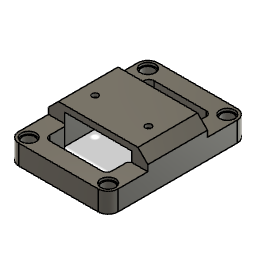
крепление двигателя (Autodesk Fusion 360 design; units mm, degrees)
Autodesk Fusion 360 part; units mm, degrees
sketch "Sketch1" plane through (0, 0, 0) normal (0, 1, 0) x (1, 0, 0)
  line L0 (-16, 24) -> (16, 24)
  line L1 (16, 24) -> (16, -24)
  line L2 (16, -24) -> (-16, -24)
  line L3 (-16, -24) -> (-16, 24)
  line L4 (-16, 24) -> (16, -24) construction
  line L5 (16, 24) -> (-16, -24) construction
  line L6 (-20, 28) -> (20, 28)
  line L7 (20, 28) -> (20, -28)
  line L8 (20, -28) -> (-20, -28)
  line L9 (-20, -28) -> (-20, 28)
  line L10 (-20, 28) -> (20, -28) construction
  line L11 (20, 28) -> (-20, -28) construction
  circle A0 centre (-16, 24) radius 2.5
  circle A1 centre (16, 24) radius 2.5
  circle A2 centre (-16, -24) radius 2.5
  circle A3 centre (16, -24) radius 2.5
  circle A4 centre (16, 24) radius 4
  circle A5 centre (-16, 24) radius 4
  circle A6 centre (-16, -24) radius 4
  circle A7 centre (16, -24) radius 4
  dimension "d1" = 32
  dimension "d2" = 48
  dimension "d3" = 40
  dimension "d4" = 56
  dimension "d5" = 5
  dimension "d6" = 5
  dimension "d7" = 5
  dimension "d8" = 5
  constraint horizontal L0
  constraint perpendicular L0 L1
  constraint parallel L0 L2
  constraint parallel L1 L3
  constraint coincident L4 origin
  constraint coincident L5 origin
  constraint horizontal L6
  constraint perpendicular L6 L7
  constraint parallel L6 L8
  constraint parallel L7 L9
  constraint coincident L10 origin
  constraint coincident L11 origin
  constraint coincident L0.start L3.end
  constraint coincident L0.end L1.start
  constraint coincident L2.end L3.start
  constraint coincident L1.end L2.start
  constraint concentric A1 A4
  constraint tangent L6 A4
  constraint concentric A0 A5
  constraint tangent L6 A5
  constraint concentric A2 A6
  constraint tangent L9 A6
  constraint concentric A3 A7
  constraint tangent L7 A7
  measures "d1" distance of L1.end L2.end
  measures "d2" distance of L0.end L1.end
  measures "d3" distance of L7.end L8.end
  measures "d4" distance of L6.end L7.end
  measures "d5" diameter of A0
  measures "d6" diameter of A1
  measures "d7" diameter of A2
  measures "d8" diameter of A3
extrude "Extrude1" add sketch "Sketch1" along normal blind 2.5 contours L0 L3 A0 A5 | L0 L3 A0 A5 | L0 L6 A4 A5 | L0 L1 L2 L3 A4 A5 A6 A7 | L3 L9 A5 A6 | L0 L1 A1 A4 | L0 L1 A1 A4 | L2 L3 A2 A6 | L2 L3 A2 A6 | L1 L7 A4 A7 | L2 L8 A6 A7 | L1 L2 A3 A7 | L1 L2 A3 A7 makes body 1
sketch "Sketch2" plane through (0, 2.5, 0) normal (0, 1, 0) x (-1, 0, 0)
  circle A0 centre (16, 24) radius 2.5
  circle A1 centre (-16, -24) radius 2.5
  circle A2 centre (-16, 24) radius 2.5
  circle A3 centre (16, -24) radius 2.5
  arc A4 (16, -28) -> (20, -24) centre (16, -24) ccw
  line L0 (20, -24) -> (20, 24)
  arc A5 (20, 24) -> (16, 28) centre (16, 24) ccw
  line L1 (16, 28) -> (-16, 28)
  arc A6 (-16, 28) -> (-20, 24) centre (-16, 24) ccw
  line L2 (-20, 24) -> (-20, -24)
  arc A7 (-20, -24) -> (-16, -28) centre (-16, -24) ccw
  line L3 (-16, -28) -> (16, -28)
  circle A8 centre (16, -24) radius 4
  circle A9 centre (-16, -24) radius 4
  circle A10 centre (-16, 24) radius 4
  circle A11 centre (16, 24) radius 4
  constraint concentric A3 A8
  constraint concentric A1 A9
  constraint concentric A2 A10
  constraint concentric A0 A11
extrude "Extrude2" add sketch "Sketch2" along normal blind 8 contours A4 A8 | A7 A9 | A5 A11 | A6 A10 bodies 1
sketch "Sketch3" plane through (0, 10.5, 0) normal (0, 1, 0) x (-1, 0, 0)
  circle A0 centre (16, -24) radius 2.5
  circle A1 centre (16, -24) radius 4
  circle A2 centre (16, -24) radius 3
  circle A3 centre (-16, -24) radius 3
  circle A4 centre (16, 24) radius 3
  circle A5 centre (-16, 24) radius 3
  dimension "d13" = 6
  dimension "d14" = 6
  dimension "d15" = 6
  dimension "d16" = 6
  constraint concentric A0 A2
  measures "d13" diameter of A2
  measures "d14" diameter of A3
  measures "d15" diameter of A4
  measures "d16" diameter of A5
extrude "Extrude3" cut sketch "Sketch3" against normal blind 1 contours A2 | A3 | A4 | A5 bodies 1
sketch "Sketch4" plane through (0, 2.5, 0) normal (0, 1, 0) x (-1, 0, 0)
  arc A0 (-20, 24) -> (-16, 28) centre (-16, 24) ccw
  line L0 (-20, 24) -> (-20, -24)
  arc A1 (-16, -28) -> (-20, -24) centre (-16, -24) ccw
  line L1 (-16, -28) -> (16, -28)
  arc A2 (20, -24) -> (16, -28) centre (16, -24) ccw
  line L2 (20, -24) -> (20, 24)
  arc A3 (16, 28) -> (20, 24) centre (16, 24) ccw
  line L3 (16, 28) -> (-16, 28)
  line L4 (12.5, -21) -> (-12.5, -21)
  line L5 (-12.5, -21) -> (-12.5, 21)
  line L6 (-12.5, 21) -> (12.5, 21)
  line L7 (12.5, 21) -> (12.5, -21)
  line L8 (12.5, -21) -> (-12.5, 21) construction
  line L9 (-12.5, -21) -> (12.5, 21) construction
  dimension "d19" = 25
  dimension "d20" = 42
  constraint horizontal L4
  constraint perpendicular L4 L5
  constraint parallel L4 L6
  constraint parallel L5 L7
  constraint coincident L8 origin
  constraint coincident L9 origin
  measures "d19" distance of L5.end L6.end
  measures "d20" distance of L4.end L5.end
extrude "Extrude4" cut sketch "Sketch4" against normal blind 16 contours L4 L5 L6 L7 bodies 1
fillet "Fillet1" radius 2 4 edges at (12.5, 1.25, -21) (-12.5, 1.25, -21) (-12.5, 1.25, 21) (12.5, 1.25, 21) on bodies 1
sketch "Sketch5" plane through (12.5, 0, 0) normal (-1, 0, 0) x (0, 0, 1)
  line L0 (19, 0) -> (19, 2.5)
  line L1 (19, 2.5) -> (-19, 2.5)
  line L2 (-19, 2.5) -> (-19, 0)
  line L3 (-19, 0) -> (19, 0)
  line L4 (0, 0) -> (0, 2.5)
  line L5 (-13, 2.5) -> (13, 2.5)
  line L6 (13, 2.5) -> (13, 0)
  line L7 (13, 0) -> (-13, 0)
  line L8 (-13, 0) -> (-13, 2.5)
  line L9 (-13, 2.5) -> (13, 0) construction
  line L10 (13, 2.5) -> (-13, 0) construction
  point P0 (0, 1.25)
  dimension "d25" = 26
  constraint coincident L4.start origin
  constraint midpoint L1 L4.end
  constraint horizontal L5
  constraint perpendicular L5 L6
  constraint parallel L5 L7
  constraint parallel L6 L8
  constraint coincident L9 P0
  constraint coincident L10 P0
  constraint midpoint L4 P0
  measures "d25" distance of L6.end L7.end
extrude "Extrude5" cut sketch "Sketch5" along normal blind -1 and the other way blind -26 contours L1 L3 L4 L5 L6 L7 | L1 L3 L4 L5 L7 L8 bodies 1
chamfer "Chamfer1" distance 1 angle 45 4 edges at (13.5, 1.25, 13) (13.5, 1.25, -13) (-13.5, 1.25, -13) (-13.5, 1.25, 13) on bodies 1
sketch "Sketch6" plane through (0, 2.5, 0) normal (0, 1, 0) x (-1, 0, 0)
  arc A0 (-20, 24) -> (-16, 28) centre (-16, 24) ccw
  line L0 (-20, 24) -> (-20, -24)
  arc A1 (-16, -28) -> (-20, -24) centre (-16, -24) ccw
  line L1 (-16, -28) -> (16, -28)
  arc A2 (20, -24) -> (16, -28) centre (16, -24) ccw
  line L2 (20, -24) -> (20, 24)
  arc A3 (16, 28) -> (20, 24) centre (16, 24) ccw
  line L3 (16, 28) -> (-16, 28)
  line L4 (-12.5, -13) -> (-13.5, -12)
  line L5 (-13.5, -12) -> (-13.5, 12)
  line L6 (-13.5, 12) -> (-12.5, 13)
  line L7 (-12.5, 13) -> (-12.5, 19)
  arc A4 (-10.5, 21) -> (-12.5, 19) centre (-10.5, 19) ccw
  line L8 (-10.5, 21) -> (10.5, 21)
  arc A5 (12.5, 19) -> (10.5, 21) centre (10.5, 19) ccw
  line L9 (12.5, 19) -> (12.5, 13)
  line L10 (12.5, 13) -> (13.5, 12)
  line L11 (13.5, 12) -> (13.5, -12)
  line L12 (13.5, -12) -> (12.5, -13)
  line L13 (12.5, -13) -> (12.5, -19)
  arc A6 (10.5, -21) -> (12.5, -19) centre (10.5, -19) ccw
  line L14 (10.5, -21) -> (-10.5, -21)
  arc A7 (-12.5, -19) -> (-10.5, -21) centre (-10.5, -19) ccw
  line L15 (-12.5, -19) -> (-12.5, -13)
  line L16 (-13.5, 12) -> (-20, 12)
  line L17 (-20, 12) -> (-20, -12)
  line L18 (-20, -12) -> (-13.5, -12)
  line L19 (-13.5, -12) -> (-13.5, 12)
  line L20 (13.5, 12) -> (20, 12)
  line L21 (20, 12) -> (20, -12)
  line L22 (20, -12) -> (13.5, -12)
  line L23 (13.5, -12) -> (13.5, 12)
  constraint horizontal L16
  constraint vertical L17
  constraint horizontal L18
  constraint vertical L19
  constraint coincident L0 L17.end
  constraint coincident L5.end L6.start
  constraint horizontal L20
  constraint vertical L21
  constraint horizontal L22
  constraint vertical L23
  constraint coincident L2 L21.end
  constraint coincident L10.end L11.start
extrude "Extrude6" add sketch "Sketch6" along normal blind 11 contours L0 L5 L16 L17 L18 L19 | L2 L11 L20 L21 L22 L23 bodies 1
extrude "Extrude7" add 2 faces at (17.8333, 13.5, 4) (-17.8333, 13.5, -4) along direction (0, 1, 0) blind 1 on bodies 1 bodies 1
sketch "Sketch7" plane through (0, 14.5, 0) normal (0, 1, 0) x (-1, 0, 0)
  line L0 (-13.5, -12) -> (-13.5, 12)
  line L1 (-13.5, 12) -> (-20, 12)
  line L2 (-20, 12) -> (-20, -12)
  line L3 (-20, -12) -> (-13.5, -12)
  line L4 (-20, 12) -> (20, 12)
  line L5 (20, 12) -> (20, -12)
  line L6 (20, -12) -> (-20, -12)
  line L7 (-20, -12) -> (-20, 12)
  dimension "d35" = 40
  constraint horizontal L4
  constraint vertical L5
  constraint horizontal L6
  constraint vertical L7
  constraint coincident L1.end L2.start
  measures "d35" distance of L1.end L4.end
extrude "Extrude8" add sketch "Sketch7" along normal blind 2.5 bodies 1
chamfer "Chamfer2" distance 4 angle 45 2 edges at (-20, 17, 0) (20, 17, 0) on bodies 1
sketch "Sketch8" plane through (0, 17, 0) normal (0, 1, 0) x (-1, 0, 0)
  line L0 (-16, 12) -> (-16, -12)
  line L1 (-16, -12) -> (16, -12)
  line L2 (16, -12) -> (16, 12)
  line L3 (16, 12) -> (-16, 12)
  line L4 (0, -12) -> (0, -3)
  line L5 (0, -3) -> (0, 8)
  line L6 (0, 2.5) -> (-10.75, 2.5)
  line L7 (-10.75, 2.5) -> (10.75, 2.5)
  circle A0 centre (-10.75, 2.5) radius 1.25
  circle A1 centre (10.75, 2.5) radius 1.25
  dimension "d39" = 9
  dimension "d40" = 11
  dimension "d41" = 10.75
  dimension "d42" = 21.5
  dimension "d43" = 2.5
  dimension "d44" = 2.5
  constraint midpoint L1 L4.start
  constraint perpendicular L1 L4
  constraint parallel L4 L5
  constraint midpoint L5 L6.start
  constraint perpendicular L5 L6
  constraint perpendicular L5 L7
  constraint coincident L6.end L7.start
  constraint coincident L7.end A1.centre
  measures "d39" distance of L4.start L4.end
  measures "d40" distance of L4.end L5.end
  measures "d41" distance of L6.start L6.end
  measures "d42" distance of L6.end L7.end
  measures "d43" diameter of A0
  measures "d44" diameter of A1
extrude "Extrude9" cut sketch "Sketch8" against normal blind 8 contours A0 | A1 bodies 1
chamfer "Chamfer3" distance 1 angle 45 2 edges at (-9.5846, 14.5, 2.048) (11.9154, 14.5, 2.048) on bodies 1
extrude "Extrude10" add 2 faces at (-16.6307, 2.5, 14.6732) (-16.6307, 2.5, -14.6732) along direction (0, 1, 0) blind 8 on bodies 1 bodies 1
copy_body "Body->Comp1" bodies 1 removing the originals makes body 2 in component "Component'"
extrude "Extrude1'" cut 1 faces at (-17.8333, 0, -4.0001) along direction (0, 1, 0) blind 2.5 on bodies 2 bodies 2 in component "Component'"
component "Component'" placed x (1, 0, 0) y (0, 1, 0) z (0, 0, 1) at (0, 0, 0)
equation "d41 = ( 21.5 / 2 ) * 1 mm"
